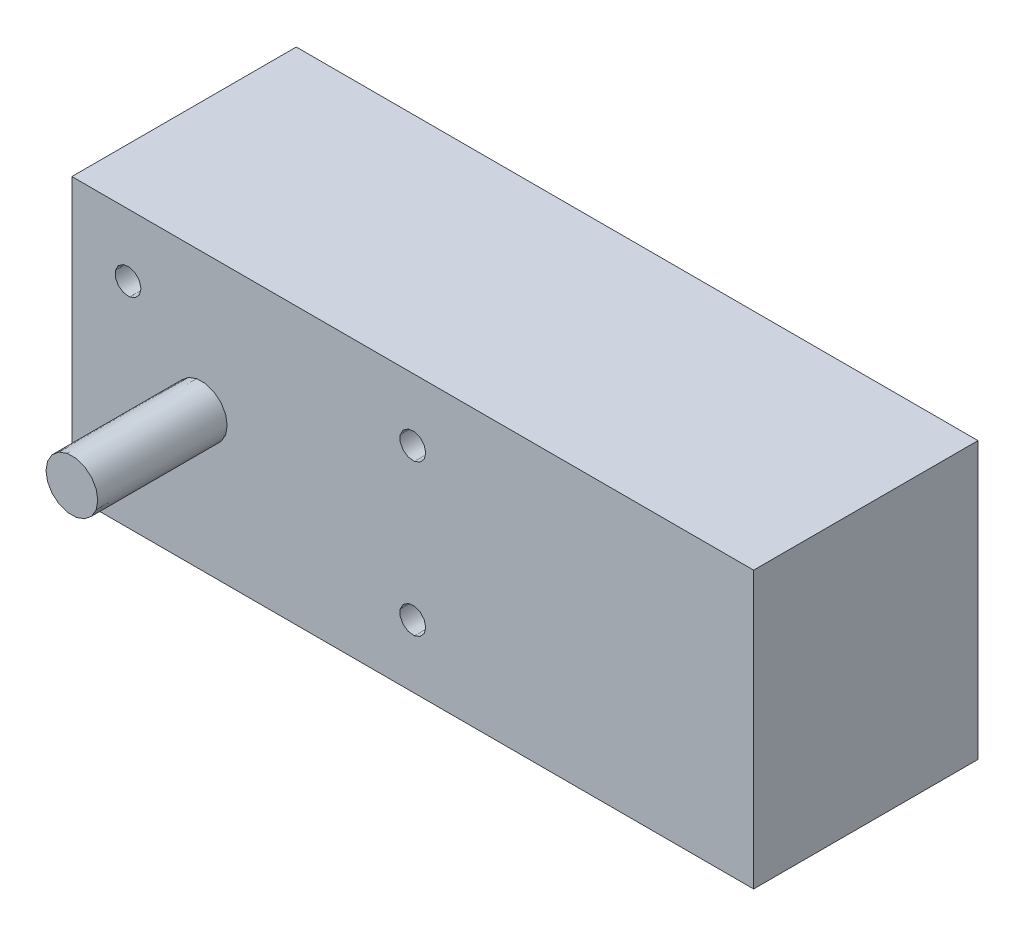
# Autodesk Inventor part: Motor
Saved by Autodesk Inventor 2017 (Build 210142000, 142)
## iProperties
Created: 2019-07-01
Part Number: Motor
Material: Generic
Document SubType Name: Modeling
Designer: Dell
Density: 1 g/cm^3
Appearance: Default
Author: Dell
Autodesk Inventor part; units mm, degrees
ref_plane "YZ Plane" through (0, 0, 0) normal (1, 0, 0) x (0, 1, 0)
ref_plane "XZ Plane" through (0, 0, 0) normal (0, 1, 0) x (-1, 0, 0)
ref_plane "XY Plane" through (0, 0, 0) normal (0, 0, 1) x (1, 0, 0)
sketch "Sketch1" plane through (0, 0, 0) normal (0, 0, 1) x (1, 0, 0)
  line L0 (0, 0) -> (79, 0)
  line L1 (79, 0) -> (79, 32)
  line L2 (79, 32) -> (0, 32)
  line L3 (0, 32) -> (0, 0)
  dimension "d0" = 79
  dimension "d1" = 32
  constraints: 8 end point, 2 parallel, 1 horizontal, 1 perpendicular
  measures "d0" distance of L2.end L1.end
  measures "d1" distance of L1.end L0.end
extrude "Extrusion1" add sketch "Sketch1" along normal blind 26
sketch "Sketch2" plane through (0, 0, 26) normal (0, 0, 1) x (1, 0, 0)
  circle A0 centre (15, 16) radius 3
  line L0 (0, 32) -> (0, 0) projected
  line L1 (6.5, 24.75) -> (39.5, 24.75) construction
  line L2 (39.5, 24.75) -> (39.5, 7.25) construction
  line L3 (39.5, 7.25) -> (6.5, 7.25) construction
  line L4 (6.5, 7.25) -> (6.5, 24.75) construction
  circle A1 centre (6.5, 24.75) radius 1.5
  circle A2 centre (6.5, 7.25) radius 1.5
  circle A3 centre (39.5, 24.75) radius 1.5
  circle A4 centre (39.5, 7.25) radius 1.5
  point P0 (0, 16)
  point P1 (6.5, 16)
  dimension "d4" = 6
  dimension "d5" = 15
  dimension "d6" = 33
  dimension "d7" = 17.5
  dimension "d8" = 8.5
  dimension "d9" = 3
  dimension "d10" = 3
  dimension "d11" = 3
  dimension "d12" = 3
  constraints: 8 end point, 5 centre point, 4 coincident, 2 horizontal alignment, 2 midpoint, 2 parallel, 1 horizontal, 1 perpendicular
  measures "d4" diameter of A0
  measures "d5" distance from line of L0 A0.centre
  measures "d6" distance of L1.start L1.end
  measures "d7" distance of L1.end L2.end
  measures "d8" distance from line of A0.centre L4
  measures "d9" diameter of A1
  measures "d10" diameter of A2
  measures "d11" diameter of A3
  measures "d12" diameter of A4
extrude "Extrusion2" add sketch "Sketch2" along normal blind 15 contours A0
extrude "Extrusion3" cut sketch "Sketch2" against normal blind 10 contours A1 | A2 | A3 | A4
body "Solid1"
